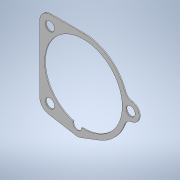
# Autodesk Inventor part: 65. Прокладка крышки подшипника
Saved by Autodesk Inventor 2021 (Build 250183000, 183)
## iProperties
Created: 2021-03-10
Part Number: 65. Прокладка крышки подшипника
Material: Типовые
Document SubType Name: Modeling
Designer: Данил
Density: 1 g/cm^3
Appearance: По умолчанию
Author: Данил
Autodesk Inventor part; units mm, degrees
ref_plane "YZ Plane" through (0, 0, 0) normal (1, 0, 0) x (0, 1, 0)
ref_plane "XZ Plane" through (0, 0, 0) normal (0, 1, 0) x (-1, 0, 0)
ref_plane "XY Plane" through (0, 0, 0) normal (0, 0, 1) x (1, 0, 0)
sketch "Эскиз1" plane through (0, 0, 0) normal (0, 0, 1) x (1, 0, 0)
  circle A0 centre (0, 0) radius 54 construction
  circle A1 centre (54, 0) radius 5.25
  arc A2 (55.3148, -9.9132) -> (55.3148, 9.9132) centre (54, 0) ccw
  arc A3 (55.3148, -9.9132) -> (47.1914, -16.522) centre (56.6296, -19.8264) ccw
  arc A4 (47.1914, 16.522) -> (55.3148, 9.9132) centre (56.6296, 19.8264) ccw
  arc A5 (17.8584, -46.702) -> (47.1914, -16.522) centre (0, 0) ccw
  arc A6 (-2.0396, -44.4532) -> (-11.7971, -42.9078) centre (0, 0) ccw
  circle A7 centre (0, 0) radius 45 construction
  line L0 (17.8584, -46.702) -> (-3.1107, -54.7204)
  line L1 (0, 0) -> (-7.0396, -44.446) construction
  line L2 (0, 0) -> (0, -45) construction
  arc A8 (-11.7971, -42.9078) -> (-2.0396, -44.4532) centre (-7.0396, -44.446) ccw
  arc A9 (-8.9301, -55.2823) -> (-3.1107, -54.7204) centre (-7.0396, -44.446) ccw
  arc A10 (47.1914, 16.522) -> (0, 50) centre (0, 0) ccw
  line L3 (0, 0) -> (-38.1838, -38.1838) construction
  line L4 (0, 0) -> (-54, 0) construction
  circle A11 centre (-38.1838, -38.1838) radius 5.25
  line L5 (-8.9301, -55.2823) -> (-40.2146, -49.8242)
  arc A12 (-50, -38.1838) -> (-40.2146, -49.8242) centre (-38.1838, -38.1838) ccw
  line L6 (-50, -38.1838) -> (-50, 38.1838)
  line L7 (0, 0) -> (-38.1838, 38.1838) construction
  circle A13 centre (-38.1838, 38.1838) radius 5.25
  arc A14 (-38.1838, 50) -> (-50, 38.1838) centre (-38.1838, 38.1838) ccw
  line L8 (-38.1838, 50) -> (0, 50)
  dimension "d0" = 108
  dimension "d1" = 10.5
  dimension "d2" = 10
  dimension "d3" = 10
  dimension "d4" = 10
  dimension "d5" = 50
  dimension "d6" = 89
  dimension "d7" = 90
  dimension "d10" = 9
  dimension "d11" = 5
  dimension "d12" = 11
  dimension "d13" = 50
  dimension "d14" = 45
  dimension "d15" = 10.5
  dimension "d16" = 90
  dimension "d17" = 10.5
  constraints: 26 point on circle, 18 end point, 15 centre point, 12 coincident, 11 tangent, 2 vertical, 1 horizontal, 1 horizontal alignment, 1 perpendicular, 1 vertical alignment
  measures "d0" diameter of A0
  measures "d1" diameter of A1
  measures "d2" radius of A2
  measures "d3" radius of A3
  measures "d4" radius of A4
  measures "d5" radius of A5
  measures "d6" diameter of A6
  measures "d7" diameter of A7
  measures "d10" angle of L1 L2
  measures "d11" radius of A8
  measures "d12" radius of A9
  measures "d13" radius of A10
  measures "d14" angle of L3 L4
  measures "d15" diameter of A11
  measures "d16" angle of L3 L7
  measures "d17" diameter of A13
extrude "Выдавливание1" add sketch "Эскиз1" along normal mid plane 1
